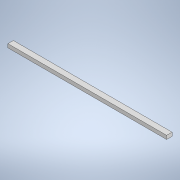
# Autodesk Inventor part: Linear_Rail_Basic
Saved by Autodesk Inventor 2021 (Build 250183000, 183)
## iProperties
Created: 2021-03-29
Part Number: Linear_Rail_Basic
Material: Generic
Document SubType Name: Modeling
Designer: Ariel Wolle
Density: 1 g/cm^3
Appearance: Default
Author: Ariel Wolle
Autodesk Inventor part; units mm, degrees
ref_plane "YZ Plane" through (0, 0, 0) normal (1, 0, 0) x (0, 1, 0)
ref_plane "XZ Plane" through (0, 0, 0) normal (0, 1, 0) x (-1, 0, 0)
ref_plane "XY Plane" through (0, 0, 0) normal (0, 0, 1) x (1, 0, 0)
sketch "Sketch1" plane through (0, 0, 0) normal (1, 0, 0) x (0, 1, 0)
  line L0 (0, 0) -> (8, 0)
  line L1 (8, 0) -> (8, -12)
  line L2 (8, -12) -> (0, -12)
  line L3 (0, -12) -> (0, 0)
  dimension "d0" = 12
  dimension "d1" = 8
  constraints: 8 end point, 2 parallel, 1 horizontal, 1 perpendicular
  measures "d0" distance of L0.end L1.end
  measures "d1" distance of L1.end L2.end
extrude "Extrusion1" add sketch "Sketch1" along normal blind 350
body "Solid1"
